Autodesk Fusion 360 part; units mm, degrees
(part 2 of 4)
  line L201 (202.55, -22.075) -> (202.55, -35.075)
  line L202 (31.6, -21.575) -> (44.6, -21.575)
  line L203 (235.6, -22.075) -> (235.6, -35.075)
  line L204 (7.7875, -21.575) -> (20.7875, -21.575)
  arc A196 (258.262, -4.025) -> (257.762, -3.525) centre (257.762, -4.025) ccw
  line L205 (69.7, -21.575) -> (82.7, -21.575)
  line L206 (107.8, -35.575) -> (120.8, -35.575)
  line L207 (21.2875, -22.075) -> (21.2875, -35.075)
  arc A197 (273.7, -3.025) -> (273.2, -2.525) centre (273.2, -3.025) ccw
  arc A198 (251.262, -18.025) -> (251.762, -18.525) centre (251.762, -18.025) ccw
  arc A199 (260.2, -2.525) -> (259.7, -3.025) centre (260.2, -3.025) ccw
  line L208 (275.638, -18.525) -> (281.638, -18.525)
  arc A200 (7.7875, -21.575) -> (7.2875, -22.075) centre (7.7875, -22.075) ccw
  line L209 (259.7, -3.025) -> (259.7, -16.025)
  line L210 (7.7875, -35.575) -> (20.7875, -35.575)
  arc A201 (63.65, -35.575) -> (64.15, -35.075) centre (63.65, -35.075) ccw
  arc A202 (7.2875, -35.075) -> (7.7875, -35.575) centre (7.7875, -35.075) ccw
  arc A203 (257.762, -18.525) -> (258.262, -18.025) centre (257.762, -18.025) ccw
  arc A204 (275.638, -3.525) -> (275.138, -4.025) centre (275.638, -4.025) ccw
  line L211 (251.262, -4.025) -> (251.262, -18.025)
  line L212 (69.7, -35.575) -> (82.7, -35.575)
  arc A205 (281.638, -18.525) -> (282.138, -18.025) centre (281.638, -18.025) ccw
  arc A206 (31.6, -21.575) -> (31.1, -22.075) centre (31.6, -22.075) ccw
  line L213 (126.85, -35.575) -> (139.85, -35.575)
  arc A207 (178.45, -22.075) -> (177.95, -21.575) centre (177.95, -22.075) ccw
  line L214 (183.5, -22.075) -> (183.5, -35.075)
  line L215 (164.95, -21.575) -> (177.95, -21.575)
  arc A208 (145.9, -21.575) -> (145.4, -22.075) centre (145.9, -22.075) ccw
  arc A209 (139.85, -35.575) -> (140.35, -35.075) centre (139.85, -35.075) ccw
  line L216 (159.4, -22.075) -> (159.4, -35.075)
  arc A210 (216.55, -22.075) -> (216.05, -21.575) centre (216.05, -22.075) ccw
  arc A211 (177.95, -35.575) -> (178.45, -35.075) centre (177.95, -35.075) ccw
  arc A212 (120.8, -35.575) -> (121.3, -35.075) centre (120.8, -35.075) ccw
  line L217 (221.6, -22.075) -> (221.6, -35.075)
  arc A213 (203.05, -21.575) -> (202.55, -22.075) centre (203.05, -22.075) ccw
  arc A214 (202.55, -35.075) -> (203.05, -35.575) centre (203.05, -35.075) ccw
  line L218 (240.65, -22.075) -> (240.65, -35.075)
  line L219 (241.15, -21.575) -> (254.15, -21.575)
  arc A215 (36.3625, -40.625) -> (35.8625, -41.125) centre (36.3625, -41.125) ccw
  arc A216 (49.3625, -54.625) -> (49.8625, -54.125) centre (49.3625, -54.125) ccw
  arc A217 (140.35, -22.075) -> (139.85, -21.575) centre (139.85, -22.075) ccw
  arc A218 (288.775, -21.575) -> (288.275, -22.075) centre (288.775, -22.075) ccw
  arc A219 (54.9125, -54.125) -> (55.4125, -54.625) centre (55.4125, -54.125) ccw
  line L220 (288.775, -35.575) -> (301.775, -35.575)
  line L221 (302.275, -22.075) -> (302.275, -35.075)
  line L222 (145.9, -35.575) -> (158.9, -35.575)
  line L223 (254.65, -22.075) -> (254.65, -35.075)
  line L224 (126.35, -22.075) -> (126.35, -35.075)
  line L225 (264.9625, -35.575) -> (277.9625, -35.575)
  line L226 (164.45, -22.075) -> (164.45, -35.075)
  arc A220 (9.6687, -54.125) -> (10.1687, -54.625) centre (10.1687, -54.125) ccw
  line L227 (222.1, -21.575) -> (235.1, -21.575)
  line L228 (68.9125, -41.125) -> (68.9125, -54.125)
  arc A221 (184, -21.575) -> (183.5, -22.075) centre (184, -22.075) ccw
  line L229 (126.85, -21.575) -> (139.85, -21.575)
  arc A222 (121.3, -22.075) -> (120.8, -21.575) centre (120.8, -22.075) ccw
  line L230 (9.6687, -41.125) -> (9.6687, -54.125)
  arc A223 (254.65, -22.075) -> (254.15, -21.575) centre (254.15, -22.075) ccw
  line L231 (145.9, -21.575) -> (158.9, -21.575)
  arc A224 (221.6, -35.075) -> (222.1, -35.575) centre (222.1, -35.075) ccw
  arc A225 (107.8, -21.575) -> (107.3, -22.075) centre (107.8, -22.075) ccw
  arc A226 (158.9, -35.575) -> (159.4, -35.075) centre (158.9, -35.075) ccw
  arc A227 (240.65, -35.075) -> (241.15, -35.575) centre (241.15, -35.075) ccw
  line L232 (107.0125, -41.125) -> (107.0125, -54.125)
  line L233 (112.0625, -41.125) -> (112.0625, -54.125)
  arc A228 (254.15, -35.575) -> (254.65, -35.075) centre (254.15, -35.075) ccw
  line L234 (121.3, -22.075) -> (121.3, -35.075)
  line L235 (107.3, -22.075) -> (107.3, -35.075)
  arc A229 (164.95, -21.575) -> (164.45, -22.075) centre (164.95, -22.075) ccw
  arc A230 (241.15, -21.575) -> (240.65, -22.075) centre (241.15, -22.075) ccw
  arc A231 (126.85, -21.575) -> (126.35, -22.075) centre (126.85, -22.075) ccw
  line L236 (203.05, -35.575) -> (216.05, -35.575)
  arc A232 (235.6, -22.075) -> (235.1, -21.575) centre (235.1, -22.075) ccw
  arc A233 (197.5, -22.075) -> (197, -21.575) centre (197, -22.075) ccw
  line L237 (216.55, -22.075) -> (216.55, -35.075)
  arc A234 (216.05, -35.575) -> (216.55, -35.075) centre (216.05, -35.075) ccw
  line L238 (264.9625, -21.575) -> (277.9625, -21.575)
  arc A235 (235.1, -35.575) -> (235.6, -35.075) centre (235.1, -35.075) ccw
  line L239 (197.5, -22.075) -> (197.5, -35.075)
  line L240 (164.95, -35.575) -> (177.95, -35.575)
  line L241 (241.15, -35.575) -> (254.15, -35.575)
  arc A236 (183.5, -35.075) -> (184, -35.575) centre (184, -35.075) ccw
  line L242 (203.05, -21.575) -> (216.05, -21.575)
  arc A237 (107.3, -35.075) -> (107.8, -35.575) centre (107.8, -35.075) ccw
  line L243 (178.45, -22.075) -> (178.45, -35.075)
  arc A238 (159.4, -22.075) -> (158.9, -21.575) centre (158.9, -22.075) ccw
  arc A239 (145.4, -35.075) -> (145.9, -35.575) centre (145.9, -35.075) ccw
  line L244 (55.4125, -54.625) -> (68.4125, -54.625)
  line L245 (55.4125, -40.625) -> (68.4125, -40.625)
  arc A240 (68.4125, -54.625) -> (68.9125, -54.125) centre (68.4125, -54.125) ccw
  line L246 (93.0125, -41.125) -> (93.0125, -54.125)
  arc A241 (93.0125, -54.125) -> (93.5125, -54.625) centre (93.5125, -54.125) ccw
  arc A242 (257.3188, -54.125) -> (257.8188, -54.625) centre (257.8188, -54.125) ccw
  arc A243 (257.8188, -40.625) -> (257.3188, -41.125) centre (257.8188, -41.125) ccw
  line L247 (131.6125, -40.625) -> (144.6125, -40.625)
  line L248 (207.3125, -41.125) -> (207.3125, -54.125)
  arc A244 (207.3125, -54.125) -> (207.8125, -54.625) centre (207.8125, -54.125) ccw
  arc A245 (131.1125, -54.125) -> (131.6125, -54.625) centre (131.6125, -54.125) ccw
  arc A246 (125.5625, -54.625) -> (126.0625, -54.125) centre (125.5625, -54.125) ccw
  line L249 (36.3625, -54.625) -> (49.3625, -54.625)
  arc A247 (264.9625, -21.575) -> (264.4625, -22.075) centre (264.9625, -22.075) ccw
  line L250 (23.6687, -41.125) -> (23.6687, -54.125)
  line L251 (288.775, -21.575) -> (301.775, -21.575)
  arc A248 (264.4625, -35.075) -> (264.9625, -35.575) centre (264.9625, -35.075) ccw
  line L252 (87.9625, -41.125) -> (87.9625, -54.125)
  arc A249 (23.1687, -54.625) -> (23.6687, -54.125) centre (23.1687, -54.125) ccw
  line L253 (35.8625, -41.125) -> (35.8625, -54.125)
  line L254 (126.0625, -41.125) -> (126.0625, -54.125)
  arc A250 (302.275, -22.075) -> (301.775, -21.575) centre (301.775, -22.075) ccw
  line L255 (93.5125, -54.625) -> (106.5125, -54.625)
  arc A251 (68.9125, -41.125) -> (68.4125, -40.625) centre (68.4125, -41.125) ccw
  arc A252 (49.8625, -41.125) -> (49.3625, -40.625) centre (49.3625, -41.125) ccw
  line L256 (188.7625, -54.625) -> (201.7625, -54.625)
  line L257 (112.5625, -54.625) -> (125.5625, -54.625)
  line L258 (74.4625, -54.625) -> (87.4625, -54.625)
  arc A253 (270.8188, -54.625) -> (271.3188, -54.125) centre (270.8188, -54.125) ccw
  arc A254 (107.0125, -41.125) -> (106.5125, -40.625) centre (106.5125, -41.125) ccw
  line L259 (10.1687, -40.625) -> (23.1687, -40.625)
  line L260 (278.4625, -22.075) -> (278.4625, -35.075)
  line L261 (74.4625, -40.625) -> (87.4625, -40.625)
  line L262 (36.3625, -40.625) -> (49.3625, -40.625)
  arc A255 (87.4625, -54.625) -> (87.9625, -54.125) centre (87.4625, -54.125) ccw
  arc A256 (126.0625, -41.125) -> (125.5625, -40.625) centre (125.5625, -41.125) ccw
  arc A257 (301.775, -35.575) -> (302.275, -35.075) centre (301.775, -35.075) ccw
  line L263 (279.7568, -42.125) -> (279.7568, -56.125)
  line L264 (93.5125, -40.625) -> (106.5125, -40.625)
  arc A258 (273.2568, -41.625) -> (272.7568, -42.125) centre (273.2568, -42.125) ccw
  line L265 (164.1625, -41.125) -> (164.1625, -54.125)
  line L266 (273.2568, -41.625) -> (279.2568, -41.625)
  arc A259 (112.5625, -40.625) -> (112.0625, -41.125) centre (112.5625, -41.125) ccw
  line L267 (112.5625, -40.625) -> (125.5625, -40.625)
  arc A260 (93.5125, -40.625) -> (93.0125, -41.125) centre (93.5125, -41.125) ccw
  line L268 (73.9625, -41.125) -> (73.9625, -54.125)
  line L269 (10.1687, -54.625) -> (23.1687, -54.625)
  arc A261 (288.275, -35.075) -> (288.775, -35.575) centre (288.775, -35.075) ccw
  line L270 (131.6125, -54.625) -> (144.6125, -54.625)
  arc A262 (73.9625, -54.125) -> (74.4625, -54.625) centre (74.4625, -54.125) ccw
  arc A263 (23.6687, -41.125) -> (23.1687, -40.625) centre (23.1687, -41.125) ccw
  line L271 (54.9125, -41.125) -> (54.9125, -54.125)
  arc A264 (87.9625, -41.125) -> (87.4625, -40.625) centre (87.4625, -41.125) ccw
  arc A265 (35.8625, -54.125) -> (36.3625, -54.625) centre (36.3625, -54.125) ccw
  arc A266 (277.9625, -35.575) -> (278.4625, -35.075) centre (277.9625, -35.075) ccw
  arc A267 (10.1687, -40.625) -> (9.6688, -41.125) centre (10.1687, -41.125) ccw
  line L272 (264.4625, -22.075) -> (264.4625, -35.075)
  line L273 (288.275, -22.075) -> (288.275, -35.075)
  arc A268 (112.0625, -54.125) -> (112.5625, -54.625) centre (112.5625, -54.125) ccw
  arc A269 (55.4125, -40.625) -> (54.9125, -41.125) centre (55.4125, -41.125) ccw
  arc A270 (106.5125, -54.625) -> (107.0125, -54.125) centre (106.5125, -54.125) ccw
  arc A271 (278.4625, -22.075) -> (277.9625, -21.575) centre (277.9625, -22.075) ccw
  line L274 (49.8625, -41.125) -> (49.8625, -54.125)
  arc A272 (74.4625, -40.625) -> (73.9625, -41.125) centre (74.4625, -41.125) ccw
  arc A273 (164.1625, -41.125) -> (163.6625, -40.625) centre (163.6625, -41.125) ccw
  arc A274 (221.3125, -41.125) -> (220.8125, -40.625) centre (220.8125, -41.125) ccw
  line L275 (207.8125, -54.625) -> (220.8125, -54.625)
  line L276 (150.1625, -41.125) -> (150.1625, -54.125)
  arc A275 (202.2625, -41.125) -> (201.7625, -40.625) centre (201.7625, -41.125) ccw
  line L277 (145.1125, -41.125) -> (145.1125, -54.125)
  arc A276 (150.1625, -54.125) -> (150.6625, -54.625) centre (150.6625, -54.125) ccw
  arc A277 (188.2625, -54.125) -> (188.7625, -54.625) centre (188.7625, -54.125) ccw
  arc A278 (169.2125, -54.125) -> (169.7125, -54.625) centre (169.7125, -54.125) ccw
  line L278 (272.7568, -42.125) -> (272.7568, -56.125)
  arc A279 (163.6625, -54.625) -> (164.1625, -54.125) centre (163.6625, -54.125) ccw
  line L279 (273.2568, -56.625) -> (279.2568, -56.625)
  arc A280 (169.7125, -40.625) -> (169.2125, -41.125) centre (169.7125, -41.125) ccw
  arc A281 (150.6625, -40.625) -> (150.1625, -41.125) centre (150.6625, -41.125) ccw
  line L280 (207.8125, -40.625) -> (220.8125, -40.625)
  arc A282 (240.3625, -41.125) -> (239.8625, -40.625) centre (239.8625, -41.125) ccw
  arc A283 (183.2125, -41.125) -> (182.7125, -40.625) centre (182.7125, -41.125) ccw
  line L281 (221.3125, -41.125) -> (221.3125, -54.125)
  line L282 (226.8625, -54.625) -> (239.8625, -54.625)
  arc A284 (271.3188, -41.125) -> (270.8188, -40.625) centre (270.8188, -41.125) ccw
  line L283 (150.6625, -54.625) -> (163.6625, -54.625)
  line L284 (257.3188, -41.125) -> (257.3188, -54.125)
  line L285 (226.3625, -41.125) -> (226.3625, -54.125)
  line L286 (169.2125, -41.125) -> (169.2125, -54.125)
  arc A285 (201.7625, -54.625) -> (202.2625, -54.125) centre (201.7625, -54.125) ccw
  arc A286 (188.7625, -40.625) -> (188.2625, -41.125) centre (188.7625, -41.125) ccw
  line L287 (257.8188, -40.625) -> (270.8188, -40.625)
  line L288 (183.2125, -41.125) -> (183.2125, -54.125)
  arc A287 (144.6125, -54.625) -> (145.1125, -54.125) centre (144.6125, -54.125) ccw
  line L289 (150.6625, -40.625) -> (163.6625, -40.625)
  line L290 (169.7125, -54.625) -> (182.7125, -54.625)
  arc A288 (207.8125, -40.625) -> (207.3125, -41.125) centre (207.8125, -41.125) ccw
  arc A289 (182.7125, -54.625) -> (183.2125, -54.125) centre (182.7125, -54.125) ccw
  arc A290 (220.8125, -54.625) -> (221.3125, -54.125) centre (220.8125, -54.125) ccw
  line L291 (188.2625, -41.125) -> (188.2625, -54.125)
  arc A291 (226.3625, -54.125) -> (226.8625, -54.625) centre (226.8625, -54.125) ccw
  line L292 (169.7125, -40.625) -> (182.7125, -40.625)
  line L293 (240.3625, -41.125) -> (240.3625, -54.125)
  line L294 (271.3188, -41.125) -> (271.3188, -54.125)
  line L295 (257.8188, -54.625) -> (270.8188, -54.625)
  arc A292 (131.6125, -40.625) -> (131.1125, -41.125) centre (131.6125, -41.125) ccw
  arc A293 (226.8625, -40.625) -> (226.3625, -41.125) centre (226.8625, -41.125) ccw
  line L296 (202.2625, -41.125) -> (202.2625, -54.125)
  arc A294 (145.1125, -41.125) -> (144.6125, -40.625) centre (144.6125, -41.125) ccw
  line L297 (226.8625, -40.625) -> (239.8625, -40.625)
  arc A295 (239.8625, -54.625) -> (240.3625, -54.125) centre (239.8625, -54.125) ccw
  line L298 (131.1125, -41.125) -> (131.1125, -54.125)
  line L299 (188.7625, -40.625) -> (201.7625, -40.625)
  line L300 (-7, -102.25) -> (311.8, -102.25)
  line L301 (311.8, 7) -> (311.8, -102.25)
  line L302 (-7, 7) -> (311.8, 7)
  line L303 (-7, 7) -> (-7, -102.25)
  arc A296 (16.025, -16.525) -> (16.525, -16.025) centre (16.025, -16.025) ccw
  line L304 (16.525, -3.025) -> (16.525, -16.025)
  arc A297 (16.525, -3.025) -> (16.025, -2.525) centre (16.025, -3.025) ccw
  line L305 (3.025, -2.525) -> (16.025, -2.525)
  arc A298 (3.025, -2.525) -> (2.525, -3.025) centre (3.025, -3.025) ccw
  line L306 (2.525, -3.025) -> (2.525, -16.025)
  arc A299 (2.525, -16.025) -> (3.025, -16.525) centre (3.025, -16.025) ccw
  line L307 (3.025, -16.525) -> (16.025, -16.525)
  dimension "d70" = -7
  dimension "d130" = 0
extrude "拉伸1" add sketch "草图5" sketch "草图4" along normal blind 8 contours L10 L12 L13 L22 | L16 L17 L20 L21 of sketch 2 makes body 1 at (299.195, 0, 410.0797) makes body 2 at (248.3947, 0, 486.2807) makes body 3 at (210.2954, 0, 372.2972)
move_body "移动1" bodies 1 2 to x (1, 0, 0) y (0, 1, 0) z (0, 0, 1) at (0, 0, -125)
combine "合并1" operation add target body 3 tool bodies 1 2
extrude "拉伸2" add sketch "草图3" along normal blind 1.5 separate body makes body 4
extrude "拉伸3" add sketch "草图2" along normal blind 8 separate body makes body 5
extrude "拉伸4" add sketch "草图1" along normal blind 3 separate body makes body 6
sketch "草图6" plane through (0, 0, 0) normal (0, -1, 0) x (1, 0, 0)
  line L0 (0.0951, -109.619) -> (318.896, -109.619)
  line L1 (318.896, -109.619) -> (318.896, -0.3693)
  line L2 (318.896, -0.3693) -> (0.0951, -0.3693)
  line L3 (0.0951, -0.3693) -> (0.0951, -109.619)
  line L4 (318.896, -109.619) -> (298.896, -109.619)
  line L5 (0.0951, -109.619) -> (20.0951, -109.619)
  line L6 (20.0951, -109.619) -> (20.0951, -84.619)
  line L7 (20.0951, -84.619) -> (20.0951, -89.619)
  line L8 (20.0951, -89.619) -> (20.0951, -94.619)
  line L9 (20.0951, -94.619) -> (20.0951, -99.619)
  line L10 (20.0951, -84.619) -> (298.896, -84.619)
  line L11 (298.896, -84.619) -> (298.896, -109.619)
  line L12 (298.896, -109.619) -> (20.0951, -109.619)
  line L13 (20.0951, -109.619) -> (20.0951, -84.619)
  line L14 (20.0951, -89.619) -> (298.896, -89.619)
  line L15 (298.896, -89.619) -> (298.896, -109.619)
  line L16 (298.896, -109.619) -> (20.0951, -109.619)
  line L17 (20.0951, -109.619) -> (20.0951, -89.619)
  line L18 (20.0951, -94.619) -> (298.896, -94.619)
  line L19 (298.896, -94.619) -> (298.896, -109.619)
  line L20 (298.896, -109.619) -> (20.0951, -109.619)
  line L21 (20.0951, -109.619) -> (20.0951, -94.619)
  line L22 (20.0951, -99.619) -> (298.896, -99.619)
  line L23 (298.896, -99.619) -> (298.896, -109.619)
  line L24 (298.896, -109.619) -> (20.0951, -109.619)
  line L25 (20.0951, -109.619) -> (20.0951, -99.619)
  dimension "d9" = 20
  dimension "d10" = 20
  dimension "d11" = 25
  dimension "d12" = 5
  dimension "d13" = 5
  dimension "d14" = 5
  constraint coincident L0.end L1.start
  constraint perpendicular L1 L4
  constraint coincident L0.start L3.end
  constraint perpendicular L3 L5
  constraint perpendicular L0 L6
  constraint perpendicular L0 L7
  constraint perpendicular L0 L8
  constraint parallel L6 L9
  constraint horizontal L10
  constraint vertical L11
  constraint horizontal L12
  constraint vertical L13
  constraint horizontal L14
  constraint vertical L15
  constraint horizontal L16
  constraint vertical L17
  constraint horizontal L18
  constraint vertical L19
  constraint horizontal L20
  constraint vertical L21
  constraint horizontal L22
  constraint vertical L23
  constraint horizontal L24
  constraint vertical L25
  measures "d9" distance of L0.end L4.end
  measures "d10" distance of L0.start L5.end
  measures "d11" distance of L5.end L6.end
  measures "d12" distance of L6.end L7.end
  measures "d13" distance of L7.end L8.end
  measures "d14" distance of L8.end L9.end
extrude "拉伸5" add sketch "草图6" along normal blind 3 separate body contours L0 L6 L11 L12 L13 L15 L16 L17 L19 L20 L21 L22 L23 L24 L25 | L6 L9 L11 L13 L15 L17 L18 L19 L21 L22 | L6 L8 L11 L13 L14 L15 L17 L18 | L6 L7 L10 L11 L13 L14 makes body 7
extrude "拉伸6" add sketch "草图6" along normal blind 3 separate body contours L0 L6 L11 L12 L13 L15 L16 L17 L19 L20 L21 L22 L23 L24 L25 | L6 L9 L11 L13 L15 L17 L18 L19 L21 L22 | L6 L8 L11 L13 L14 L15 L17 L18 makes body 8
extrude "拉伸7" add sketch "草图6" along normal blind 3 separate body contours L0 L6 L11 L12 L13 L15 L16 L17 L19 L20 L21 L22 L23 L24 L25 | L6 L9 L11 L13 L15 L17 L18 L19 L21 L22 makes body 9
extrude "拉伸8" add sketch "草图6" along normal blind 3 separate body contours L0 L6 L11 L12 L13 L15 L16 L17 L19 L20 L21 L22 L23 L24 L25 makes body 10
extrude "拉伸19" add sketch "草图25" along normal blind 1.5 separate body contours L28 L31 L32 L35 | L300 L301 L302 L303 makes body 11
extrude "拉伸20" cut 1 faces at (-13.2, 0.5, 179.4167) along direction (-1, 0, 0) blind 0.03 on bodies 11 bodies 11
extrude "拉伸21" cut 1 faces at (-225.7433, 0.5, 143) along direction (0, 0, 1) blind 0.03 on bodies 11 bodies 11
extrude "拉伸22" cut 1 faces at (-332, 1, 179.4367) along direction (1, 0, 0) blind 0.03 on bodies 11 bodies 11
extrude "拉伸23" cut 1 faces at (-225.7233, 0.5, 252.25) along direction (0, 0, -1) blind 0.03 on bodies 11 bodies 11
move_body "移动2" bodies 8 9 10 to x (1, 0, 0) y (0, 1, 0) z (0, 0, 1) at (0, -3, 0)
move_body "移动3" bodies 9 10 to x (1, 0, 0) y (0, 1, 0) z (0, 0, 1) at (0, -3, 0)
move_body "移动4" bodies 10 to x (1, 0, 0) y (0, 1, 0) z (0, 0, 1) at (0, -3, 0)
move_body "移动5" bodies 5 to x (1, 0, 0) y (0, 1, 0) z (0, 0, 1) at (0, 3, -125)
move_body "移动6" bodies 4 to x (1, 0, 0) y (0, 1, 0) z (0, 0, 1) at (0, 13, -250)
move_body "移动7" bodies 3 to x (1, 0, 0) y (0, 1, 0) z (0, 0, 1) at (0, 14.5, -375)
move_body "移动9" bodies 3 4 to x (1, 0, 0) y (0, 1, 0) z (0, 0, 1) at (0, -2, 0)
move_body "移动12" bodies 11 to x (1, 0, 0) y (0, 1, 0) z (0, 0, 1) at (290, 0, -261)
move_body "移动13" bodies 11 to x (1, 0, 0) y (0, 1, 0) z (0, 0, 1) at (42.0651, 11, 8.4107)
extrude "拉伸27" add 1 faces at (318.8351, 11.5, -73.1626) along direction (1, 0, 0) blind 0.061 separate body on bodies 11 makes body 12
extrude "拉伸28" add 1 faces at (106.3418, 11.5, -109.5593) along direction (0, 0, -1) blind 0.06 separate body on bodies 11 makes body 13
extrude "拉伸29" add 1 faces at (318.8554, 11.5, -109.5593) along direction (0, 0, -1) blind 0.06 separate body on bodies 12 makes body 14
combine "合并5" operation add target body 13 tool bodies 14 12 11
sketch "草图8" plane through (0, 20.5, 0) normal (0, 1, 0) x (-1, 0, 0)
  line L0 (-318.896, -0.3693) -> (-318.896, -109.619)
  line L1 (-318.896, -109.619) -> (-0.0951, -109.619)
  line L2 (-0.0951, -109.619) -> (-0.0951, -0.3693)
  line L3 (-0.0951, -0.3693) -> (-318.896, -0.3693)
  line L4 (-292.845, -102.62) -> (-292.845, -83.5699)
  line L5 (-292.845, -83.5699) -> (-311.895, -83.5699)
  line L6 (-311.895, -83.5699) -> (-311.895, -7.3697)
  line L7 (-311.895, -7.3697) -> (-254.744, -7.3697)
  line L8 (-254.744, -7.3697) -> (-254.744, -26.4184)
  line L9 (-254.744, -26.4184) -> (-245.22, -26.4184)
  line L10 (-245.22, -26.4184) -> (-245.22, -7.3697)
  line L11 (-245.22, -7.3697) -> (-7.0942, -7.3697)
  line L12 (-7.0941, -7.3697) -> (-7.0941, -102.62)
  line L13 (-7.0941, -102.62) -> (-292.845, -102.62)
  line L14 (-7.0941, -102.62) -> (-7.0941, -106.12)
  line L15 (-292.845, -102.62) -> (-311.895, -102.62)
  line L16 (-311.895, -102.62) -> (-311.895, -106.12)
  line L17 (-311.895, -106.12) -> (-210.895, -106.12)
  line L18 (-210.895, -106.12) -> (-109.895, -106.12)
  line L19 (-109.895, -106.12) -> (-7.0941, -106.12)
  line L20 (-311.895, -7.3697) -> (-311.895, -3.8697)
  line L21 (-311.895, -3.8697) -> (-210.895, -3.8697)
  line L22 (-210.895, -3.8697) -> (-109.895, -3.8697)
  line L23 (-109.895, -3.8697) -> (-7.0941, -3.8697)
  point P0 (-109.895, -106.12)
  point P1 (-210.895, -106.12)
  point P2 (-311.895, -102.62)
  point P3 (-311.895, -106.12)
  point P4 (-311.895, -3.8697)
  point P5 (-210.895, -3.8697)
  point P6 (-109.895, -3.8697)
  point P7 (-7.0941, -3.8697)
  dimension "d27" = 3.5
  dimension "d28" = 3.5
  dimension "d29" = 101
  dimension "d30" = 101
  dimension "d31" = 3.5
  dimension "d32" = 101
  dimension "d33" = 101
  constraint coincident L12.end L13.start
  constraint perpendicular L1 L14
  constraint coincident L4.start L13.end
  constraint perpendicular L4 L15
  constraint perpendicular L1 L16
  constraint perpendicular L2 L17
  constraint perpendicular L2 L18
  constraint perpendicular L14 L19
  constraint coincident L6.end L7.start
  constraint perpendicular L7 L20
  constraint perpendicular L10 L21
  constraint perpendicular L10 L22
  constraint perpendicular L2 L23
  constraint coincident P0 L18.end
  constraint coincident P1 L17.end
  constraint coincident P2 L15.end
  constraint coincident P3 L16.end
  constraint coincident P4 L20.end
  constraint coincident P5 L21.end
  constraint coincident P6 L22.end
  constraint coincident P7 L23.end
  measures "d27" distance of L12.end L14.end
  measures "d28" distance of P2 P3
  measures "d29" distance of P3 P1
  measures "d30" distance of P1 P0
  measures "d31" distance of L6.end P4
  measures "d32" distance of P4 P5
  measures "d33" distance of P5 P6
hole "孔1" at (7.0941, 20.5, -106.12) at (109.895, 20.5, -106.12) at (109.895, 20.5, -3.8697) at (7.0941, 20.5, -3.8697) at (210.895, 20.5, -106.12) at (210.895, 20.5, -3.8697) at (311.895, 20.5, -106.12) at (311.895, 20.5, -3.8697) direction (0, -1, 0) diameter 2.2 depth 40 tip angle 180 bodies 3 4 5 6 7 8 9 10 13
hole "孔2" at (109.895, 20.5, -106.12) at (210.895, 20.5, -106.12) direction (0, -1, 0) diameter 3.4 depth 40 tip angle 180 bodies 4 5 6 7 8 9
hole "孔3" at (7.0941, 20.5, -106.12) at (7.0941, 20.5, -3.8697) at (109.895, 20.5, -3.8697) at (210.895, 20.5, -3.8697) at (311.895, 20.5, -3.8697) at (311.895, 20.5, -106.12) direction (0, -1, 0) diameter 3.4 depth 40 tip angle 180 bodies 4 5 13
extrude "拉伸13" cut 1 faces at (292.845, 15.1667, -89.9199) along direction (1, 0, 0) blind 0.2 on bodies 3 bodies 3
extrude "拉伸14" cut 1 faces at (305.6117, 17.8333, -83.5699) along direction (0, 0, -1) blind 0.2 on bodies 3 bodies 3
extrude "拉伸15" cut 1 faces at (245.22, 15.1667, -13.7193) along direction (1, 0, 0) blind 0.2 on bodies 3 bodies 3
extrude "拉伸16" cut 1 faces at (254.744, 15.1667, -20.0688) along direction (-1, 0, 0) blind 0.2 on bodies 3 bodies 3
fillet "圆角1" radius 3 32 edges at (318.896, 16.5, -0.3693) (318.896, 16.5, -109.619) (0.0951, 16.5, -109.619) (0.0951, 16.5, -0.3693) (318.896, 11.75, -0.3693) (318.896, 11.75, -109.619) (0.0951, 11.75, -109.619) (0.0951, 11.75, -0.3693) (318.896, 7, -0.3693) (318.896, 7, -109.619) (0.0951, 7, -109.619) (0.0951, 7, -0.3693) (318.896, 1.5, -0.3693) (318.896, 1.5, -109.619) (0.0951, 1.5, -109.619) (0.0951, 1.5, -0.3693) (298.896, -1.5, -84.619) (298.896, -1.5, -109.619) (20.0951, -1.5, -109.619) (20.0951, -1.5, -84.619) (298.896, -4.5, -89.619) (298.896, -4.5, -109.619) (20.0951, -4.5, -109.619) (20.0951, -4.5, -89.619) (298.896, -7.5, -94.619) (298.896, -7.5, -109.619) (20.0951, -7.5, -109.619) (20.0951, -7.5, -94.619) (298.896, -10.5, -99.619) (298.896, -10.5, -109.619) (20.0951, -10.5, -109.619) (20.0951, -10.5, -99.619) on bodies 3 4 5 6 7 8 9 10
fillet "圆角1" radius 1.5 3 edges at (311.895, 16.5, -7.3697) (7.0941, 16.5, -102.62) (7.0941, 16.5, -7.3697) on bodies 3 4 5 6 7 8 9 10
fillet "圆角1" radius 1.5 7 edges at (293.045, 16.5, -102.62) (293.045, 16.5, -83.7699) (311.895, 16.5, -83.7699) (254.544, 16.5, -7.3697) (254.544, 16.5, -26.4184) (245.42, 16.5, -26.4184) (245.42, 16.5, -7.3697) on bodies 3 4 5 6 7 8 9 10
fillet "圆角5" radius 3 4 edges at (0.0951, 11.75, -109.6193) (0.0951, 11.75, -0.3693) (318.8961, 11.75, -0.3693) (318.8961, 11.75, -109.6193) on bodies 13
sketch "草图21" plane through (0, 20.5, 0) normal (0, 1, 0) x (-1, 0, 0)
  line L0 (-311.895, -82.2699) -> (-311.895, -8.8697)
  arc A0 (-310.395, -7.3697) -> (-311.895, -8.8697) centre (-310.395, -8.8697) ccw
  line L1 (-243.92, -7.3697) -> (-8.5942, -7.3697)
  line L2 (-253.044, -26.4184) -> (-246.92, -26.4184)
  arc A1 (-7.0942, -8.8697) -> (-8.5942, -7.3697) centre (-8.5942, -8.8697) ccw
  line L3 (-7.0942, -8.8697) -> (-7.0942, -101.12)
  arc A2 (-8.5942, -102.62) -> (-7.0941, -101.12) centre (-8.5942, -101.12) ccw
  line L4 (-8.5942, -102.62) -> (-291.545, -102.62)
  arc A3 (-0.0951, -3.3693) -> (-3.0951, -0.3693) centre (-3.0951, -3.3693) ccw
  line L5 (-3.0951, -0.3693) -> (-315.896, -0.3693)
  arc A4 (-315.896, -0.3693) -> (-318.896, -3.3693) centre (-315.896, -3.3693) ccw
  line L6 (-318.896, -3.3693) -> (-318.896, -106.619)
  arc A5 (-318.896, -106.619) -> (-315.896, -109.619) centre (-315.896, -106.619) ccw
  line L7 (-315.896, -109.619) -> (-3.0951, -109.619)
  arc A6 (-3.0951, -109.619) -> (-0.0951, -106.619) centre (-3.0951, -106.619) ccw
  line L8 (-0.0951, -106.619) -> (-0.0951, -3.3693)
  circle A7 centre (-311.895, -3.8697) radius 1.1
  circle A8 centre (-210.895, -3.8697) radius 1.1
  circle A9 centre (-7.0941, -3.8697) radius 1.1
  circle A10 centre (-109.895, -106.12) radius 1.1
  circle A11 centre (-7.0941, -106.12) radius 1.1
  circle A12 centre (-109.895, -3.8697) radius 1.1
  circle A13 centre (-210.895, -106.12) radius 1.1
  circle A14 centre (-311.895, -106.12) radius 1.1
  line L9 (-294.345, -85.0699) -> (-310.345, -85.0699)
  line L10 (-310.345, -85.0699) -> (-310.345, -101.0699)
  line L11 (-310.345, -101.0699) -> (-294.345, -101.0699)
  line L12 (-294.345, -101.0699) -> (-294.345, -85.0699)
  line L13 (-254.544, -8.8697) -> (-254.544, -24.9184)
  line L14 (-245.42, -24.9184) -> (-245.42, -8.8697)
  line L15 (-293.045, -101.12) -> (-293.045, -85.2699)
  line L16 (-294.545, -83.7699) -> (-310.395, -83.7699)
  line L17 (-310.395, -7.3697) -> (-256.044, -7.3697)
  arc A15 (-246.92, -26.4184) -> (-245.42, -24.9184) centre (-246.92, -24.9184) ccw
  arc A16 (-243.92, -7.3697) -> (-245.42, -8.8697) centre (-243.92, -8.8697) ccw
  arc A17 (-293.045, -101.12) -> (-291.545, -102.62) centre (-291.545, -101.12) ccw
  arc A18 (-293.045, -85.2699) -> (-294.545, -83.7699) centre (-294.545, -85.2699) ccw
  arc A19 (-311.895, -82.2699) -> (-310.395, -83.7699) centre (-310.395, -82.2699) ccw
  arc A20 (-254.544, -8.8697) -> (-256.044, -7.3697) centre (-256.044, -8.8697) ccw
  arc A21 (-254.544, -24.9184) -> (-253.044, -26.4184) centre (-253.044, -24.9184) ccw
  dimension "d48" = 16
  dimension "d49" = 16
  constraint horizontal L9
  constraint vertical L10
  constraint horizontal L11
  constraint vertical L12
  measures "d48" distance of L9.start L9.end
  measures "d49" distance of L9.start L11.end
extrude "拉伸11" add sketch "草图21" along normal blind 3 separate body contours L9 L10 L11 L12 makes body 15
fillet "圆角2" radius 1.5 4 edges at (294.345, 22, -85.0699) (310.345, 22, -85.0699) (294.345, 22, -101.0699) (310.345, 22, -101.0699) on bodies 15
move_body "移动10" bodies 15 to x (1, 0, 0) y (0, 1, 0) z (0, 0, 1) at (1.5, 0, -1.5)
move_body "移动11" bodies 15 to x (1, 0, 0) y (0, 1, 0) z (0, 0, 1) at (0, -3, 0)
combine "合并2" operation cut target body 3 tool bodies 15 keep tools
sketch "草图22" plane through (0, 20.5, 0) normal (0, 1, 0) x (-1, 0, 0)
  arc A0 (-311.845, -101.0699) -> (-310.345, -102.5699) centre (-310.345, -101.0699) ccw
  line L0 (-310.345, -102.5699) -> (-297.345, -102.5699)
  arc A1 (-297.345, -102.5699) -> (-295.845, -101.0699) centre (-297.345, -101.0699) ccw
  line L1 (-295.845, -101.0699) -> (-295.845, -88.0699)
  arc A2 (-295.845, -88.0699) -> (-297.345, -86.5699) centre (-297.345, -88.0699) ccw
  line L2 (-297.345, -86.5699) -> (-310.345, -86.5699)
  arc A3 (-310.345, -86.5699) -> (-311.845, -88.0699) centre (-310.345, -88.0699) ccw
  line L3 (-311.845, -88.0699) -> (-311.845, -101.0699)
  spline S0 degree 3 poles (-297.6906, -95.5944) (-297.6112, -95.8921) (-298.4389, -95.8677) (-298.7383, -96.1183) knots 0 0 0 0 1 1 1 1
  spline S1 degree 3 poles (-298.7383, -96.1183) (-299.2503, -96.5469) (-299.6753, -97.5073) (-300.7624, -98.1662) knots 0 0 0 0 1 1 1 1
  spline S2 degree 3 poles (-300.7624, -98.1662) (-301.2414, -98.4565) (-301.6315, -98.702) (-302.334, -98.8329) knots 0 0 0 0 1 1 1 1
  spline S3 degree 3 poles (-302.334, -98.8329) (-302.6543, -98.8927) (-302.992, -98.8548) (-303.3103, -98.7853) knots 0 0 0 0 1 1 1 1
  spline S4 degree 3 poles (-303.3103, -98.7853) (-305.0367, -98.4083) (-305.5598, -97.8489) (-306.4774, -95.3325) knots 0 0 0 0 1 1 1 1
  spline S5 degree 3 poles (-306.4774, -95.3325) (-306.7874, -94.4823) (-307.0816, -93.4903) (-308.049, -93.1417) knots 0 0 0 0 1 1 1 1
  spline S6 degree 3 poles (-308.049, -93.1417) (-310.0362, -92.4257) (-311.1968, -94.0527) (-311.0256, -93.7847) knots 0 0 0 0 1 1 1 1
  spline S7 degree 3 poles (-311.0256, -93.7847) (-310.4126, -92.8254) (-307.3599, -89.9912) (-305.1201, -89.5699) knots 0 0 0 0 1 1 1 1
  spline S8 degree 3 poles (-305.1201, -89.5699) (-304.3708, -89.4289) (-304.0134, -89.3006) (-303.1198, -89.5222) knots 0 0 0 0 1 1 1 1
  spline S9 degree 3 poles (-303.1198, -89.5222) (-300.0901, -90.2738) (-299.6908, -93.2489) (-299.2146, -94.3324) knots 0 0 0 0 1 1 1 1
  spline S10 degree 3 poles (-299.2146, -94.3324) (-298.9491, -94.9362) (-297.7699, -95.2968) (-297.6906, -95.5944) knots 0 0 0 0 1 1 1 1
  circle A4 centre (-302.2149, -95.6421) radius 0.4286
  point P0 (-302.6436, -95.6421)
extrude "拉伸12" add sketch "草图22" along normal blind 1 contours S0 S1 S2 S3 S4 S5 S6 S7 S8 S9 S10 bodies 15
extrude "拉伸17" add 1 faces at (316.5623, 20.5, -64.0861) along direction (0, -1, 0) blind 3 separate body on bodies 3 makes body 16
combine "合并3" operation cut target body 3 tool bodies 16 keep tools
extrude "拉伸18" add 1 faces at (316.5623, 11, -39.1194) along direction (0, -1, 0) blind 3 separate body on bodies 5 makes body 17
combine "合并4" operation cut target body 5 tool bodies 17 keep tools
extrude "拉伸25" cut 2 faces at (154.495, 10, -107.286) (154.495, 4.6667, -107.286) along direction (-1, 0, 0) blind 0.5 on bodies 5 17 bodies 5 17
extrude "拉伸26" cut 2 faces at (164.495, 10, -104.953) (164.495, 4.6667, -104.953) along direction (1, 0, 0) blind 0.5 on bodies 5 17 bodies 5 17
fillet "圆角3" radius 1.5 4 edges at (153.995, 5.5, -102.62) (164.995, 5.5, -102.62) (153.995, 9.5, -102.62) (164.995, 9.5, -102.62) on bodies 5 17
fillet "圆角4" radius 1.5 8 edges at (7.0941, 5.5, -102.62) (7.0941, 5.5, -7.3697) (311.895, 5.5, -7.3697) (311.895, 5.5, -102.62) (7.0941, 9.5, -102.62) (7.0941, 9.5, -7.3697) (311.895, 9.5, -7.3697) (311.895, 9.5, -102.62) on bodies 5 17
copy_body "实体->零部件2" bodies 15 removing the originals makes body 18 in component "鸟"
sketch "草图26" plane through (0, 20.5, 0) normal (0, 1, 0) x (-1, 0, 0)
  arc A0 (-311.845, -101.0699) -> (-310.345, -102.5699) centre (-310.345, -101.0699) ccw
  line L0 (-310.345, -102.5699) -> (-297.345, -102.5699)
  arc A1 (-297.345, -102.5699) -> (-295.845, -101.0699) centre (-297.345, -101.0699) ccw
  line L1 (-295.845, -101.0699) -> (-295.845, -88.0699)
  arc A2 (-295.845, -88.0699) -> (-297.345, -86.5699) centre (-297.345, -88.0699) ccw
  line L2 (-297.345, -86.5699) -> (-310.345, -86.5699)
  arc A3 (-310.345, -86.5699) -> (-311.845, -88.0699) centre (-310.345, -88.0699) ccw
  line L3 (-311.845, -88.0699) -> (-311.845, -101.0699)
  spline S0 degree 3 poles (-299.2146, -94.3324) (-298.9491, -94.9362) (-297.7699, -95.2968) (-297.6906, -95.5944) knots 0 0 0 0 1 1 1 1
  spline S1 degree 3 poles (-297.6906, -95.5944) (-297.6112, -95.8921) (-298.4389, -95.8677) (-298.7383, -96.1183) knots 0 0 0 0 1 1 1 1
  spline S2 degree 3 poles (-298.7383, -96.1183) (-299.2503, -96.5469) (-299.6753, -97.5073) (-300.7624, -98.1662) knots 0 0 0 0 1 1 1 1
  spline S3 degree 3 poles (-300.7624, -98.1662) (-301.2414, -98.4565) (-301.6315, -98.702) (-302.334, -98.8329) knots 0 0 0 0 1 1 1 1
  spline S4 degree 3 poles (-302.334, -98.8329) (-302.6543, -98.8927) (-302.992, -98.8548) (-303.3103, -98.7853) knots 0 0 0 0 1 1 1 1
  spline S5 degree 3 poles (-303.3103, -98.7853) (-305.0367, -98.4083) (-305.5598, -97.8489) (-306.4774, -95.3325) knots 0 0 0 0 1 1 1 1
  spline S6 degree 3 poles (-306.4774, -95.3325) (-306.7874, -94.4823) (-307.0816, -93.4903) (-308.049, -93.1417) knots 0 0 0 0 1 1 1 1
  spline S7 degree 3 poles (-308.049, -93.1417) (-310.0362, -92.4257) (-311.1968, -94.0527) (-311.0256, -93.7847) knots 0 0 0 0 1 1 1 1
  spline S8 degree 3 poles (-311.0256, -93.7847) (-310.4126, -92.8254) (-307.3599, -89.9912) (-305.1201, -89.5699) knots 0 0 0 0 1 1 1 1
  spline S9 degree 3 poles (-305.1201, -89.5699) (-304.3708, -89.4289) (-304.0134, -89.3006) (-303.1198, -89.5222) knots 0 0 0 0 1 1 1 1
  spline S10 degree 3 poles (-303.1198, -89.5222) (-300.0901, -90.2738) (-299.6908, -93.2489) (-299.2146, -94.3324) knots 0 0 0 0 1 1 1 1
  line L4 (-297.345, -86.4699) -> (-310.345, -86.4699)
  arc A4 (-310.345, -86.4699) -> (-311.945, -88.0699) centre (-310.345, -88.0699) ccw
  line L5 (-311.945, -88.0699) -> (-311.945, -101.0699)
  arc A5 (-311.945, -101.0699) -> (-310.345, -102.6699) centre (-310.345, -101.0699) ccw
  line L6 (-310.345, -102.6699) -> (-297.345, -102.6699)
  arc A6 (-297.345, -102.6699) -> (-295.745, -101.0699) centre (-297.345, -101.0699) ccw
  line L7 (-295.745, -101.0699) -> (-295.745, -88.0699)
  arc A7 (-295.745, -88.0699) -> (-297.345, -86.4699) centre (-297.345, -88.0699) ccw
  dimension "d83" = 0.1
extrude "拉伸24" cut sketch "草图26" against normal blind 3 contours L4 A4 L5 A5 L6 A6 L7 A7 bodies 16
extrude "拉伸1'" cut 1 faces at (309.654, 20.5, -97.0599) along direction (0, -1, 0) blind 0.04 on bodies 18 bodies 18 in component "鸟"
sketch "草图27" plane through (0, 0, 0) normal (0, -1, 0) x (1, 0, 0)
  arc A0 (3.0951, -0.3693) -> (0.0951, -3.3693) centre (3.0951, -3.3693) ccw
  arc A1 (318.896, -3.3693) -> (315.896, -0.3693) centre (315.896, -3.3693) ccw
  line L0 (315.896, -0.3693) -> (3.0951, -0.3693)
  line L1 (0.0951, -5.8705) -> (0.0951, -3.3693)
  line L2 (315.8948, -8.9988) -> (3.0939, -8.8705)
  arc A2 (0.0951, -5.8705) -> (3.0939, -8.8705) centre (3.0951, -5.8705) ccw
  arc A3 (315.8948, -8.9988) -> (318.896, -5.9988) centre (315.896, -5.9988) ccw
  line L3 (318.896, -5.9988) -> (318.896, -3.3693)
  arc A4 (318.896, -3.3693) -> (315.896, -0.3693) centre (315.896, -3.3693) ccw
  line L4 (315.896, -0.3693) -> (3.0951, -0.3693)
  arc A5 (3.0951, -0.3693) -> (0.0951, -3.3693) centre (3.0951, -3.3693) ccw
  circle A6 centre (311.895, -3.8697) radius 1.7
  circle A7 centre (210.895, -3.8697) radius 1.7
  circle A8 centre (109.895, -3.8697) radius 1.7
  circle A9 centre (7.0941, -3.8697) radius 1.7
  dimension "d91" = 3
  dimension "d92" = 3.4
  dimension "d93" = 3.4
  dimension "d94" = 3.4
  dimension "d95" = 3.4
  constraint coincident A0.end L1.end
  constraint tangent L1 A2
  constraint tangent L2 A2
  constraint tangent L2 A3
  constraint equal A2 A3
  constraint coincident A1.start L3.end
  constraint tangent A1 L3
  constraint coincident A1.end L0.start
  constraint coincident A0.start L0.end
  constraint tangent L4 A5
  constraint tangent L1 A5
  measures "d91" radius of A2
  measures "d92" diameter of A6
  measures "d93" diameter of A7
  measures "d94" diameter of A8
  measures "d95" diameter of A9
sketch "草图40" plane through (0, 11, 0) normal (0, 1, 0) x (-1, 0, 0)
  arc A0 (-164.995, -104.12) -> (-166.495, -102.62) centre (-166.495, -104.12) ccw
  line L0 (-166.495, -102.62) -> (-310.395, -102.62)
  arc A1 (-311.895, -101.12) -> (-310.395, -102.62) centre (-310.395, -101.12) ccw
  line L1 (-311.895, -101.12) -> (-311.895, -8.8697)
  arc A2 (-310.395, -7.3697) -> (-311.895, -8.8697) centre (-310.395, -8.8697) ccw
  line L2 (-310.395, -7.3697) -> (-8.5941, -7.3697)
  arc A3 (-7.0942, -8.8697) -> (-8.5941, -7.3697) centre (-8.5942, -8.8697) ccw
  line L3 (-7.0941, -8.8697) -> (-7.0941, -101.12)
  arc A4 (-8.5942, -102.62) -> (-7.0941, -101.12) centre (-8.5942, -101.12) ccw
  line L4 (-8.5942, -102.62) -> (-152.495, -102.62)
  arc A5 (-152.495, -102.62) -> (-153.995, -104.12) centre (-152.495, -104.12) ccw
  line L5 (-153.995, -104.12) -> (-153.995, -109.619)
  line L6 (-153.995, -109.619) -> (-3.0951, -109.619)
  arc A6 (-3.0951, -109.619) -> (-0.0951, -106.619) centre (-3.0951, -106.619) ccw
  line L7 (-0.0951, -106.619) -> (-0.0951, -3.3693)
  arc A7 (-0.0951, -3.3693) -> (-3.0951, -0.3693) centre (-3.0951, -3.3693) ccw
  line L8 (-3.0951, -0.3693) -> (-315.896, -0.3693)
  arc A8 (-315.896, -0.3693) -> (-318.896, -3.3693) centre (-315.896, -3.3693) ccw
  line L9 (-318.896, -3.3693) -> (-318.896, -106.619)
  arc A9 (-318.896, -106.619) -> (-315.896, -109.619) centre (-315.896, -106.619) ccw
  line L10 (-315.896, -109.619) -> (-164.995, -109.619)
  line L11 (-164.995, -109.619) -> (-164.995, -104.12)
  circle A10 centre (-311.895, -3.8697) radius 1.7
  circle A11 centre (-109.895, -3.8697) radius 1.7
  circle A12 centre (-7.0941, -106.12) radius 1.7
  circle A13 centre (-7.0941, -3.8697) radius 1.7
  circle A14 centre (-210.895, -3.8697) radius 1.7
  circle A15 centre (-311.895, -106.12) radius 1.7
  circle A16 centre (-109.895, -106.12) radius 1.7
  circle A17 centre (-210.895, -106.12) radius 1.7
  line L12 (-164.995, -109.619) -> (-164.995, -104.12)
  line L13 (-166.495, -103.62) -> (-310.395, -103.62)
  arc A18 (-312.895, -101.12) -> (-310.395, -103.62) centre (-310.395, -101.12) ccw
  line L14 (-312.895, -101.12) -> (-312.895, -8.8697)
  arc A19 (-310.395, -6.3697) -> (-312.895, -8.8697) centre (-310.395, -8.8697) ccw
  line L15 (-310.395, -6.3697) -> (-8.5941, -6.3697)
  arc A20 (-6.0942, -8.8697) -> (-8.5941, -6.3697) centre (-8.5942, -8.8697) ccw
  line L16 (-6.0942, -8.8697) -> (-6.0941, -101.12)
  arc A21 (-8.5942, -103.62) -> (-6.0942, -101.12) centre (-8.5942, -101.12) ccw
  line L17 (-8.5942, -103.62) -> (-152.495, -103.62)
  line L18 (-153.995, -104.12) -> (-153.995, -109.619)
  line L19 (-153.995, -104.12) -> (-153.995, -104.62)
  line L20 (-152.995, -103.62) -> (-152.495, -103.62)
  line L21 (-164.995, -104.12) -> (-164.995, -104.62)
  line L22 (-165.995, -103.62) -> (-166.495, -103.62)
  line L23 (-153.995, -109.619) -> (-164.995, -109.619)
  arc A22 (-152.995, -103.62) -> (-153.995, -104.62) centre (-152.995, -104.62) ccw
  arc A23 (-164.995, -104.62) -> (-165.995, -103.62) centre (-165.995, -104.62) ccw
  dimension "d119" = 1
  dimension "d120" = 1
  constraint parallel L11 L12
  constraint parallel L0 L13
  constraint concentric A1 A18
  constraint parallel L1 L14
  constraint concentric A2 A19
  constraint parallel L2 L15
  constraint concentric A3 A20
  constraint parallel L3 L16
  constraint concentric A4 A21
  constraint parallel L4 L17
  constraint parallel L5 L18
  constraint tangent L13 A18
  constraint tangent A21 L17
  constraint tangent A19 L15
  constraint tangent A18 L14
  constraint tangent L14 A19
  constraint tangent L15 A20
  constraint tangent A20 L16
  constraint tangent L16 A21
  constraint perpendicular L17 L19
  constraint perpendicular L5 L20
  constraint perpendicular L13 L21
  constraint perpendicular L12 L22
  constraint perpendicular L12 L23
  constraint tangent L19 A22
  constraint tangent L20 A22
  constraint tangent L21 A23
  constraint tangent L22 A23
  measures "d119" radius of A22
  measures "d120" radius of A23
extrude "拉伸30" cut sketch "草图40" against normal blind 8 contours A0 L0 A1 L1 A2 L2 A3 L3 A4 L4 A5 L5 L11 L12 L13 A18 L14 A19 L15 A20 L16 A21 L17 L18 L19 L20 L21 L22 A22 A23 bodies 5 17
extrude "拉伸2'" cut 1 faces at (304.8304, 21.5, -93.0082) along direction (0, -1, 0) blind 1.04 on bodies 18 bodies 18 in component "鸟"
extrude "拉伸3'" cut 1 faces at (302.2885, 20.5, -95.7751) along direction (0, -1, 0) blind 0.04 on bodies 18 bodies 18 in component "鸟"
sketch "草图54" plane through (295.845, 20.46, -101.0699) normal (0, 1, 0) x (0, 0, 1)
  spline S0 degree 3 poles (1.7908, 11.1986) (1.7985, 10.8212) (1.2129, 10.376) (1.5622, 10.3604) knots 0 0 0 0 1 1 1 1
  spline S1 degree 3 poles (3.01, 13.1798) (2.8788, 13.1602) (2.586, 14.1048) (0.9526, 14.0942) knots 0 0 0 0 1 1 1 1
  spline S2 degree 3 poles (1.2574, 11.8844) (1.2826, 11.3764) (1.7857, 11.4476) (1.7908, 11.1986) knots 0 0 0 0 1 1 1 1
  spline S3 degree 3 poles (5.4484, 11.1986) (5.3694, 9.7062) (3.0735, 8.4889) (3.0862, 6.398) knots 0 0 0 0 1 1 1 1
  spline S4 degree 3 poles (5.8294, 1.9022) (11.1062, 1.9804) (14.392, 14.8788) (3.01, 13.1798) knots 0 0 0 0 1 1 1 1
  spline S5 degree 3 poles (0.9526, 14.0942) (0.4701, 14.0911) (1.1785, 13.6547) (1.1812, 13.637) knots 0 0 0 0 1 1 1 1
  spline S6 degree 3 poles (1.0288, 13.1036) (1.0148, 12.4428) (1.4585, 12.6227) (1.486, 12.4178) knots 0 0 0 0 1 1 1 1
  spline S7 degree 3 poles (3.0862, 6.398) (3.1005, 4.0317) (4.6459, 1.8847) (5.8294, 1.9022) knots 0 0 0 0 1 1 1 1
  spline S8 degree 3 poles (1.5622, 10.3604) (2.007, 10.3405) (3.278, 11.5359) (3.0862, 12.4178) knots 0 0 0 0 1 1 1 1
  spline S9 degree 3 poles (3.0862, 12.4178) (3.0582, 12.5464) (5.5182, 12.5179) (5.4484, 11.1986) knots 0 0 0 0 1 1 1 1
  circle A0 centre (5.3462, 4.547) radius 0.4953
  spline S10 degree 3 poles (1.1812, 13.637) (1.2221, 13.3675) (1.0359, 13.4408) (1.0288, 13.1036) knots 0 0 0 0 1 1 1 1
  spline S11 degree 3 poles (5.6008, 2.1308) (6.3554, 4.5074) (12.1984, 6.1055) (8.0392, 12.7226) knots 0 0 0 0 1 1 1 1
  spline S12 degree 3 poles (1.486, 12.4178) (1.5216, 12.1515) (1.2363, 12.3077) (1.2574, 11.8844) knots 0 0 0 0 1 1 1 1
  line L0 (8.0392, 12.7226) -> (8.0277, 12.7409)
  line L1 (5.6008, 2.1308) -> (5.5397, 1.9384)
  constraint coincident S4 L0.end
  constraint coincident S7 L1.end
extrude "拉伸4'" add sketch "草图54" along normal blind 1 contours S0 S1 S2 S3 S4 S5 S6 S7 S8 S9 S10 S11 S12 L0 L1 bodies 18 in component "鸟"
extrude "拉伸5'" add sketch "草图54" along normal blind 0.7 contours S4 S7 S11 L0 L1 | A0 bodies 18 in component "鸟"
chamfer "倒角1" distance 0.3 angle 45 3 edges at (301.6815, 21.46, -92.4072) (308.5767, 21.46, -93.0365) (297.8796, 21.46, -95.4997) on bodies 18 in component "鸟"
sketch "草图55" plane through (0, 20.5, 0) normal (0, 1, 0) x (-1, 0, 0)
  line L0 (-310.345, -86.4699) -> (-297.345, -86.4699)
  arc A0 (-295.745, -88.0699) -> (-297.345, -86.4699) centre (-297.345, -88.0699) ccw
  line L1 (-295.745, -88.0699) -> (-295.745, -101.0699)
  arc A1 (-297.345, -102.6699) -> (-295.745, -101.0699) centre (-297.345, -101.0699) ccw
  line L2 (-297.345, -102.6699) -> (-310.345, -102.6699)
  arc A2 (-311.945, -101.0699) -> (-310.345, -102.6699) centre (-310.345, -101.0699) ccw
  line L3 (-311.945, -101.0699) -> (-311.945, -88.0699)
  arc A3 (-310.345, -86.4699) -> (-311.945, -88.0699) centre (-310.345, -88.0699) ccw
  circle A4 centre (-311.895, -106.12) radius 1.1
  circle A5 centre (-210.895, -106.12) radius 1.1
  circle A6 centre (-109.895, -3.8697) radius 1.1
  circle A7 centre (-7.0941, -106.12) radius 1.1
  circle A8 centre (-109.895, -106.12) radius 1.1
  circle A9 centre (-7.0941, -3.8697) radius 1.1
  circle A10 centre (-210.895, -3.8697) radius 1.1
  circle A11 centre (-311.895, -3.8697) radius 1.1
  arc A12 (-0.0951, -3.3693) -> (-3.0951, -0.3693) centre (-3.0951, -3.3693) ccw
  line L4 (-3.0951, -0.3693) -> (-315.896, -0.3693)
  arc A13 (-315.896, -0.3693) -> (-318.896, -3.3693) centre (-315.896, -3.3693) ccw
  line L5 (-318.896, -3.3693) -> (-318.896, -106.619)
  arc A14 (-318.896, -106.619) -> (-315.896, -109.619) centre (-315.896, -106.619) ccw
  line L6 (-315.896, -109.619) -> (-3.0951, -109.619)
  arc A15 (-3.0951, -109.619) -> (-0.0951, -106.619) centre (-3.0951, -106.619) ccw
  line L7 (-0.0951, -106.619) -> (-0.0951, -3.3693)
  arc A16 (-246.92, -26.4184) -> (-245.42, -24.9184) centre (-246.92, -24.9184) ccw
  line L8 (-245.42, -24.9184) -> (-245.42, -8.8697)
  arc A17 (-243.92, -7.3697) -> (-245.42, -8.8697) centre (-243.92, -8.8697) ccw
  line L9 (-243.92, -7.3697) -> (-8.5942, -7.3697)
  arc A18 (-7.0942, -8.8697) -> (-8.5942, -7.3697) centre (-8.5942, -8.8697) ccw
  line L10 (-7.0942, -8.8697) -> (-7.0942, -101.12)
  arc A19 (-8.5941, -102.62) -> (-7.0941, -101.12) centre (-8.5942, -101.12) ccw
  line L11 (-8.5941, -102.62) -> (-291.545, -102.62)
  arc A20 (-293.045, -101.12) -> (-291.545, -102.62) centre (-291.545, -101.12) ccw
  line L12 (-293.045, -101.12) -> (-293.045, -85.2699)
  arc A21 (-293.045, -85.2699) -> (-294.545, -83.7699) centre (-294.545, -85.2699) ccw
  line L13 (-294.545, -83.7699) -> (-310.395, -83.7699)
  arc A22 (-311.895, -82.2699) -> (-310.395, -83.7699) centre (-310.395, -82.2699) ccw
  line L14 (-311.895, -82.2699) -> (-311.895, -8.8697)
  arc A23 (-310.395, -7.3697) -> (-311.895, -8.8697) centre (-310.395, -8.8697) ccw
  line L15 (-310.395, -7.3697) -> (-256.044, -7.3697)
  arc A24 (-254.544, -8.8697) -> (-256.044, -7.3697) centre (-256.044, -8.8697) ccw
  line L16 (-254.544, -8.8697) -> (-254.544, -24.9184)
  arc A25 (-254.544, -24.9184) -> (-253.044, -26.4184) centre (-253.044, -24.9184) ccw
  line L17 (-253.044, -26.4184) -> (-246.92, -26.4184)
sketch "草图56" plane through (0, 17.5, 0) normal (0, 1, 0) x (-1, 0, 0)
  arc A0 (-246.92, -26.4184) -> (-245.42, -24.9184) centre (-246.92, -24.9184) ccw
  line L0 (-245.42, -24.9184) -> (-245.42, -8.8697)
  arc A1 (-243.92, -7.3697) -> (-245.42, -8.8697) centre (-243.92, -8.8697) ccw
  line L1 (-243.92, -7.3697) -> (-8.5942, -7.3697)
  arc A2 (-7.0942, -8.8697) -> (-8.5942, -7.3697) centre (-8.5942, -8.8697) ccw
  line L2 (-7.0942, -8.8697) -> (-7.0941, -101.12)
  arc A3 (-8.5941, -102.62) -> (-7.0941, -101.12) centre (-8.5942, -101.12) ccw
  line L3 (-8.5941, -102.62) -> (-291.545, -102.62)
  arc A4 (-293.045, -101.12) -> (-291.545, -102.62) centre (-291.545, -101.12) ccw
  line L4 (-293.045, -101.12) -> (-293.045, -85.2699)
  arc A5 (-293.045, -85.2699) -> (-294.545, -83.7699) centre (-294.545, -85.2699) ccw
  line L5 (-294.545, -83.7699) -> (-310.395, -83.7699)
  arc A6 (-311.895, -82.2699) -> (-310.395, -83.7699) centre (-310.395, -82.2699) ccw
  line L6 (-311.895, -82.2699) -> (-311.895, -8.8697)
  arc A7 (-310.395, -7.3697) -> (-311.895, -8.8697) centre (-310.395, -8.8697) ccw
  line L7 (-310.395, -7.3697) -> (-256.044, -7.3697)
  arc A8 (-254.544, -8.8697) -> (-256.044, -7.3697) centre (-256.044, -8.8697) ccw
  line L8 (-254.544, -8.8697) -> (-254.544, -24.9184)
  arc A9 (-254.544, -24.9184) -> (-253.044, -26.4184) centre (-253.044, -24.9184) ccw
  line L9 (-253.044, -26.4184) -> (-246.92, -26.4184)
  arc A10 (-0.0951, -3.3693) -> (-3.0951, -0.3693) centre (-3.0951, -3.3693) ccw
  line L10 (-3.0951, -0.3693) -> (-315.896, -0.3693)
  arc A11 (-315.896, -0.3693) -> (-318.896, -3.3693) centre (-315.896, -3.3693) ccw
  line L11 (-318.896, -3.3693) -> (-318.896, -106.619)
  arc A12 (-318.896, -106.619) -> (-315.896, -109.619) centre (-315.896, -106.619) ccw
  line L12 (-315.896, -109.619) -> (-3.0951, -109.619)
  arc A13 (-3.0951, -109.619) -> (-0.0951, -106.619) centre (-3.0951, -106.619) ccw
  line L13 (-0.0951, -106.619) -> (-0.0951, -3.3693)
  circle A14 centre (-311.895, -3.8697) radius 1.1
  circle A15 centre (-210.895, -3.8697) radius 1.1
  circle A16 centre (-7.0941, -3.8697) radius 1.1
  circle A17 centre (-109.895, -106.12) radius 1.1
  circle A18 centre (-7.0941, -106.12) radius 1.1
  circle A19 centre (-109.895, -3.8697) radius 1.1
  circle A20 centre (-210.895, -106.12) radius 1.1
  circle A21 centre (-311.895, -106.12) radius 1.1